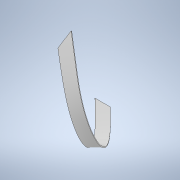
# Autodesk Inventor part: firstseatbeltpart
Saved by Autodesk Inventor 2021 (Build 250183000, 183)
## iProperties
Created: 2020-10-12
Part Number: firstseatbeltpart
Material: Generic
Document SubType Name: Modeling
Designer: atwaterh
Density: 1 g/cm^3
Appearance: Default
Author: atwaterh
Autodesk Inventor part; units mm, degrees
ref_plane "YZ Plane" through (0, 0, 0) normal (1, 0, 0) x (0, 1, 0)
ref_plane "XZ Plane" through (0, 0, 0) normal (0, 1, 0) x (-1, 0, 0)
ref_plane "XY Plane" through (0, 0, 0) normal (0, 0, 1) x (1, 0, 0)
sketch "Sketch2" plane through (0, 0, 0) normal (0, 0, 1) x (1, 0, 0)
  line L0 (0, 0) -> (0, 2.54)
  line L1 (0, 2.54) -> (50.8, 2.54)
  line L2 (50.8, 2.54) -> (50.8, 0)
  line L3 (50.8, 0) -> (0, 0)
  dimension "d12" = 2.54
  dimension "d13" = 50.8
  constraints: 8 end point, 2 perpendicular, 1 parallel, 1 vertical
  measures "d12" distance of L0.start L0.end
  measures "d13" distance of L0.end L1.end
sketch3d "3D Sketch1"
  spline S0 degree 2 poles (-69.8766, 73.0871, 92.9051) (60.6245, 6.1722, 216.0263) (-55.2126, 119.7859, 134.3128) knots 1 1 1 2 2 2
sweep "Sweep2" add profiles "Sketch2" path "3D Sketch1"
body "Solid2"
